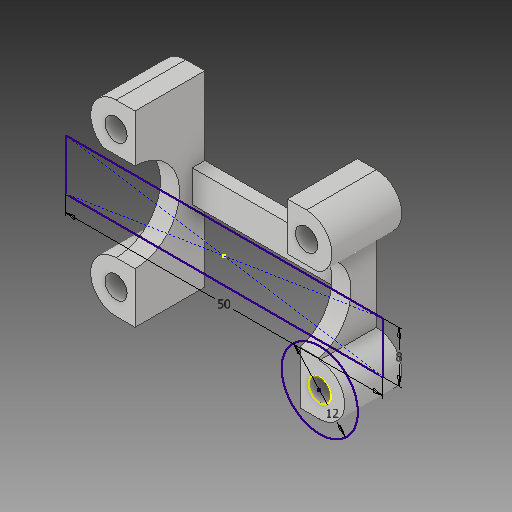
# Autodesk Inventor part: Fastening
Saved by Autodesk Inventor 2019 (Build 230136000, 136)
## iProperties
Created: 2021-07-19
Part Number: Fastening
Material: Типовые
Document SubType Name: Modeling
Designer: koryb
Density: 1 g/cm^3
Appearance: По умолчанию
Author: koryb
Autodesk Inventor part; units mm, degrees
ref_plane "YZ Plane" through (0, 0, 0) normal (1, 0, 0) x (0, 1, 0)
ref_plane "XZ Plane" through (0, 0, 0) normal (0, 1, 0) x (-1, 0, 0)
ref_plane "XY Plane" through (0, 0, 0) normal (0, 0, 1) x (1, 0, 0)
sketch "Эскиз1" plane through (0, 0, 0) normal (0, 0, 1) x (1, 0, 0)
  circle A0 centre (15, 10.75) radius 1.75 projected
  circle A1 centre (-15, 10.75) radius 1.75 projected
  circle A2 centre (-15, -10.75) radius 1.75 projected
  circle A3 centre (15, -10.75) radius 1.75 projected
  arc A4 (15, 6.75) -> (15, 14.75) centre (15, 10.75) ccw projected
  arc A5 (15, -14.75) -> (15, -6.75) centre (15, -10.75) ccw projected
  arc A6 (-15, 14.75) -> (-15, 6.75) centre (-15, 10.75) ccw projected
  arc A7 (-15, -6.75) -> (-15, -14.75) centre (-15, -10.75) ccw projected
  line L0 (15, 14.75) -> (12, 14.75)
  line L1 (12, 14.75) -> (12, -14.75)
  line L2 (12, -14.75) -> (15, -14.75)
  line L3 (15, -6.75) -> (15, 6.75)
  line L4 (-15, 14.75) -> (-12, 14.75)
  line L5 (-12, 14.75) -> (-12, -14.75)
  line L6 (-12, -14.75) -> (-15, -14.75)
  line L7 (-15, -6.75) -> (-15, 6.75)
  point P0 (0, 0)
  dimension "d0" = 3
  constraints: 16 end point, 6 perpendicular, 2 horizontal, 1 collinear
  measures "d0" distance of L0.start L0.end
extrude "Выдавливание1" add sketch "Эскиз1" along normal blind 11
sketch "Эскиз2" plane through (-12, -14.75, 0) normal (1, 0, 0) x (0, 0, -1)
  line L0 (-11, 0) -> (-11, 29.5) projected
  line L1 (-11, 29.5) -> (-5, 29.5)
  line L2 (-5, 0) -> (-11, 0)
  line L3 (-11, 0) -> (-11, 29.5)
  line L4 (0, 0) -> (-11, 0) projected
  arc A0 (-11, 8) -> (-11, 22) centre (-11, 15) ccw
  point P0 (0, 14.75)
  dimension "d4" = 6
  dimension "d5" = 7
  dimension "d13" = 14.5
  constraints: 6 end point, 3 point on line, 2 collinear, 2 point on circle, 1 centre point, 1 horizontal, 1 parallel
  measures "d4" distance of L0.end L1.end
  measures "d5" radius of A0
  measures "d13" distance of L0.end A0.centre
extrude "Выдавливание2" cut sketch "Эскиз2" along normal blind 30 and the other way blind 6
sketch "Эскиз3" plane through (0, 0, 0) normal (0, 0, -1) x (-1, 0, 0)
  line L0 (12, 14.75) -> (12, -14.75) projected
  line L1 (-12, -2.5) -> (12, -2.5)
  line L2 (12, -2.5) -> (12, 2.5)
  line L3 (12, 2.5) -> (-12, 2.5)
  line L4 (-12, 2.5) -> (-12, -2.5)
  line L5 (-12, -2.5) -> (12, 2.5) construction
  line L6 (12, -2.5) -> (-12, 2.5) construction
  point P0 (0, 0)
  dimension "d10" = 5
  constraints: 12 end point, 2 midpoint, 2 parallel, 1 horizontal, 1 perpendicular, 1 point on line
  measures "d10" distance of L2.end L1.end
extrude "Выдавливание3" add sketch "Эскиз3" against normal blind 2
sketch "Эскиз5" plane through (0, 0, 11) normal (0, 0, 1) x (1, 0, 0)
  circle A0 centre (15, -10.75) radius 1.75 projected
  line L0 (15, -6.75) -> (12, -6.75) projected
  line L1 (12, -6.75) -> (12, -14.75) projected
  line L2 (12, -14.75) -> (15, -14.75) projected
  arc A1 (15, -14.75) -> (15, -6.75) centre (15, -10.75) ccw projected
  line L3 (12, -6.75) -> (15, -6.75)
  line L4 (15, -6.75) -> (15, -2.5)
  line L5 (15, -2.5) -> (12, -2.5)
  line L6 (12, -2.5) -> (12, -6.75)
  point P0 (0, 0)
  constraints: 8 end point, 2 parallel, 1 horizontal, 1 perpendicular
extrude "Выдавливание4" cut sketch "Эскиз5" against normal blind 2
sketch "Эскиз6" plane through (0, 0, 9) normal (0, 0, 1) x (1, 0, 0)
  line L0 (-25, 4) -> (25, 4)
  line L1 (25, 4) -> (25, -4)
  line L2 (25, -4) -> (-25, -4)
  line L3 (-25, -4) -> (-25, 4)
  line L4 (-25, 4) -> (25, -4) construction
  line L5 (25, 4) -> (-25, -4) construction
  circle A0 centre (15, -10.75) radius 1.75 projected
  circle A1 centre (15, -10.75) radius 6
  point P0 (0, 0)
  dimension "d19" = 50
  dimension "d20" = 8
  dimension "d21" = 12
  constraints: 12 end point, 2 midpoint, 2 parallel, 1 centre point, 1 coincident, 1 horizontal, 1 perpendicular
  measures "d19" distance of L1.end L2.end
  measures "d20" distance of L0.end L1.end
  measures "d21" diameter of A1
